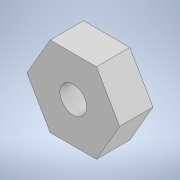
# Autodesk Inventor part: PX9200-01_Wheel_Hex
Saved by Autodesk Inventor 2022.3 (Build 263350000, 350)
## iProperties
Created: 2022-07-07
Part Number: PX9200-01_Wheel_Hex
Material: Generic
Document SubType Name: Modeling
Designer: luis_
Density: 1 g/cm^3
Appearance: Default
Author: luis_
Autodesk Inventor part; units mm, degrees
ref_plane "YZ Plane" through (0, 0, 0) normal (1, 0, 0) x (0, 1, 0)
ref_plane "XZ Plane" through (0, 0, 0) normal (0, 1, 0) x (-1, 0, 0)
ref_plane "XY Plane" through (0, 0, 0) normal (0, 0, 1) x (1, 0, 0)
sketch "Sketch1" plane through (0, 0, 0) normal (0, 0, 1) x (1, 0, 0)
  line L0 (6.9282, 0) -> (3.4641, -6)
  line L1 (3.4641, -6) -> (-3.4641, -6)
  line L2 (-3.4641, -6) -> (-6.9282, 0)
  line L3 (-6.9282, 0) -> (-3.4641, 6)
  line L4 (-3.4641, 6) -> (3.4641, 6)
  line L5 (3.4641, 6) -> (6.9282, 0)
  point P0 (0, 0)
  point P1 (0, 0)
  dimension "d0" = 12
  constraints: 12 end point, 1 coincident, 13 other
  measures "d0" distance between parallel lines of L1 L4
extrude "Extrusion1" add sketch "Sketch1" along normal blind 5
sketch "Sketch2" plane through (0, 0, 5) normal (0, 0, 1) x (1, 0, 0)
  circle A0 centre (0, 0) radius 2
  dimension "d3" = 4
  constraints: 1 centre point, 1 coincident
  measures "d3" diameter of A0
extrude "Extrusion2" cut sketch "Sketch2" against normal blind 5
body "Solid1"
